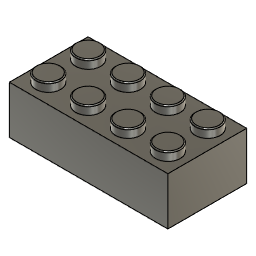
day1 lego (Autodesk Fusion 360 design; units mm, degrees)
part number: try
Autodesk Fusion 360 part; units mm, degrees
note: some values were not read from the file. Set by a fixed rule: which face or edge a step refers to.
sketch "草图1" plane through (0, 0, 0) normal (0, 0, 1) x (1, 0, 0)
  line L0 (0, 0) -> (31.8, 0)
  line L1 (31.8, 0) -> (31.8, -15.8)
  line L2 (31.8, -15.8) -> (0, -15.8)
  line L3 (0, -15.8) -> (0, 0)
  dimension "d1" = 31.8
  dimension "d2" = 15.8
  constraint horizontal L0
  constraint vertical L1
  constraint horizontal L2
  constraint vertical L3
  constraint coincident L0.start L3.end
  measures "d1" distance of L0.start L0.end
  measures "d2" distance of L0.start L2.end
extrude "拉伸1" add sketch "草图1" along normal blind 9.6
sketch "草图2" plane through (0, 0, 9.6) normal (0, 0, 1) x (-1, 0, 0)
  line L0 (0, 15.8) -> (-31.8, 15.8)
  line L1 (-31.8, 15.8) -> (-31.8, 0)
  line L2 (-31.8, 0) -> (0, 0)
  line L3 (0, 0) -> (0, 15.8)
  circle A0 centre (-3.9, 3.9) radius 2.5
  dimension "d5" = 5
  dimension "d6" = 3.9
  dimension "d7" = 3.9
  measures "d5" diameter of A0
  measures "d6" distance of L2 A0.centre
  measures "d7" distance of L3 A0.centre
extrude "拉伸2" add sketch "草图2" along normal blind 1.7 contours A0
pattern_linear "R-阵列1" count 4 spacing 8 along (1, 0, 0) count 2 spacing 8 along (0, -1, 0) of "拉伸2"
shell "抽壳1" thickness 1.49 removed faces 1 at (10.6, -10.5333, 0)
sketch "草图3" plane through (0, 0, 8.11) normal (0, 0, -1) x (1, 0, 0)
  circle A0 centre (27.9, 11.9) radius 1.01
  circle A1 centre (19.9, 11.9) radius 1.01
  circle A2 centre (11.9, 11.9) radius 1.01
  circle A3 centre (3.9, 11.9) radius 1.01
  circle A4 centre (27.9, 3.9) radius 1.01
  circle A5 centre (19.9, 3.9) radius 1.01
  circle A6 centre (11.9, 3.9) radius 1.01
  circle A7 centre (3.9, 3.9) radius 1.01
  line L0 (30.31, 14.31) -> (1.49, 14.31)
  line L1 (1.49, 14.31) -> (1.49, 1.49)
  line L2 (1.49, 1.49) -> (30.31, 1.49)
  line L3 (30.31, 1.49) -> (30.31, 14.31)
  line L4 (19.9, 3.9) -> (27.9, 11.9) construction
  circle A8 centre (23.9, 7.9) radius 3.1569
  circle A9 centre (27.9, 11.9) radius 2.5
  circle A10 centre (23.9, 7.9) radius 2.1569
  dimension "d15" = -1
  constraint coincident A5.centre L4.start
  constraint coincident A0.centre L4.end
  constraint midpoint L4 A8.centre
  constraint tangent A8 A9
extrude "拉伸3" add sketch "草图3" along normal blind 8.1 contours A8
pattern_linear "R-阵列2" count 3 spacing 8 along (-1, 0, 0) of "拉伸3"
fillet "圆角1" radius 0.2 8 faces at (3.9825, -4.4608, 11.3) (3.9825, -12.4608, 11.3) (12.0102, -4.5209, 11.3) (12.0102, -12.5209, 11.3) (20.0102, -4.5209, 11.3) (20.0102, -12.5209, 11.3) (28.0102, -4.5209, 11.3) (28.0102, -12.5209, 11.3)
fillet "圆角2" radius 0.2 3 faces at (26.7118, -8.0568, 0.01) (18.7037, -8.164, 0.01) (10.7037, -8.164, 0.01)
